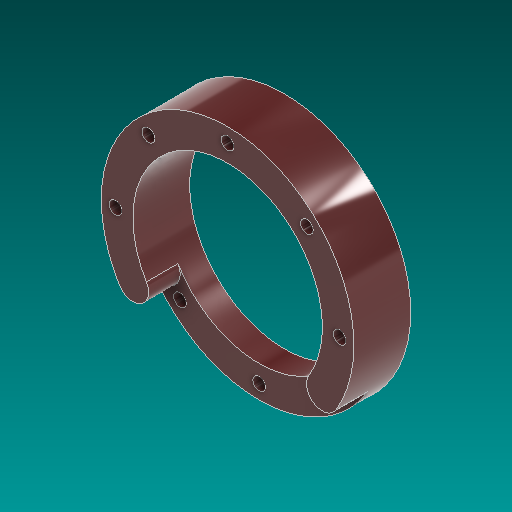
# Autodesk Inventor part: spacerVoorLager
Saved by Autodesk Inventor 2020.3 (Build 243373000, 373)
## iProperties
Created: 2020-05-24
Part Number: spacerVoorLager
Material: Generic
Document SubType Name: Modeling
Designer: Svend
Density: 1 g/cm^3
Appearance: Default
Author: Svend
Autodesk Inventor part; units mm, degrees
ref_plane "YZ Plane" through (0, 0, 0) normal (1, 0, 0) x (0, 1, 0)
ref_plane "XZ Plane" through (0, 0, 0) normal (0, 1, 0) x (-1, 0, 0)
ref_plane "XY Plane" through (0, 0, 0) normal (0, 0, 1) x (1, 0, 0)
sketch "Sketch1" plane through (0, 0, 0) normal (0, 0, 1) x (1, 0, 0)
  circle A0 centre (0, 0) radius 40
  circle A1 centre (0, 0) radius 30
  circle A2 centre (35.5, 0) radius 2
  circle A3 centre (25.1023, 25.1023) radius 2
  circle A4 centre (0, 35.5) radius 2
  circle A5 centre (-25.1023, 25.1023) radius 2
  circle A6 centre (-35.5, 0) radius 2
  circle A7 centre (-25.1023, -25.1023) radius 2
  circle A8 centre (0, -35.5) radius 2
  circle A9 centre (25.1023, -25.1023) radius 2
  dimension "d0" = 80
  dimension "d1" = 60
  dimension "d2" = 4
  dimension "d3" = 35.5
  dimension "d6" = 360
  constraints: 10 centre point, 2 coincident, 1 horizontal alignment, 17 other
  measures "d0" diameter of A0
  measures "d1" diameter of A1
  measures "d2" diameter of A2
  measures "d3" distance of point (0, 0) A2.centre
extrude "Extrusion1" add sketch "Sketch1" along normal blind 8
sketch "Sketch2" plane through (0, 0, 8) normal (0, 0, 1) x (1, 0, 0)
  circle A0 centre (0, 0) radius 40 projected
  circle A1 centre (25.1023, -25.1023) radius 2 projected
  circle A2 centre (0, -35.5) radius 2 projected
  circle A3 centre (-25.1023, -25.1023) radius 2 projected
  circle A4 centre (-35.5, 0) radius 2 projected
  circle A5 centre (-25.1023, 25.1023) radius 2 projected
  circle A6 centre (0, 35.5) radius 2 projected
  circle A7 centre (25.1023, 25.1023) radius 2 projected
  circle A8 centre (35.5, 0) radius 2 projected
  circle A9 centre (0, 0) radius 30 projected
  circle A10 centre (0, 0) radius 40 projected
  arc A11 (-34.2857, -20.6032) -> (-25.7143, -15.4524) centre (-30, -18.0278) ccw
  arc A12 (25.7143, -15.4524) -> (34.2857, -20.6032) centre (30, -18.0278) ccw
  circle A13 centre (0, 0) radius 30 projected
  circle A14 centre (0, 0) radius 40 projected
  dimension "d11" = 30
  dimension "d12" = 30
  constraints: 6 point on circle, 3 tangent, 2 centre point, 1 equal radius, 5 other
  measures "d11" horizontal distance of point (0, 0) A11.centre
  measures "d12" horizontal distance of A12.centre point (0, 0)
extrude "Extrusion2" add sketch "Sketch2" along normal blind 10 contours A0 A12 A9 A11 picked at (-33.9569, -7.8256)
equation "\"d12\" = d11"
body "Solid1"
